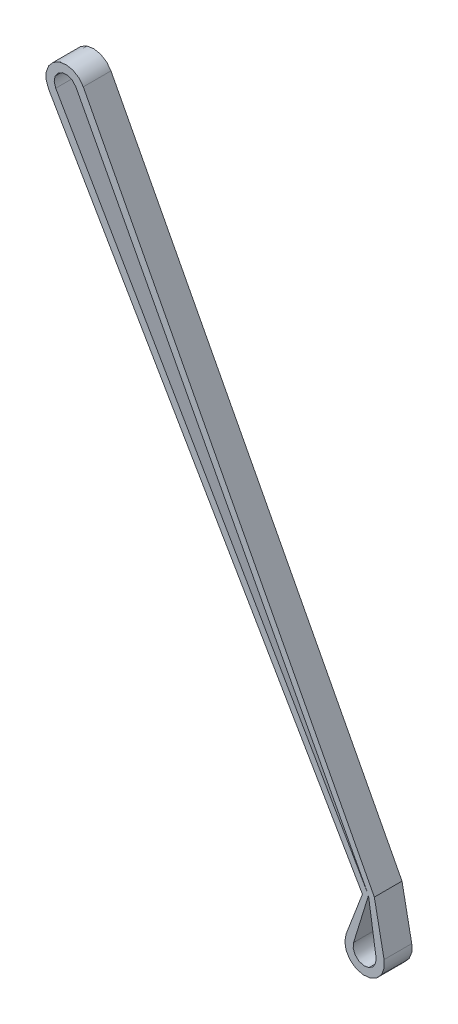
# Autodesk Inventor part: Angle Changer left band
Saved by Autodesk Inventor 2023.2 (Build 272271030, 271C)
## iProperties
Created: 2023-04-07
Part Number: Angle Changer left band
Material: Generic
Document SubType Name: Modeling
Designer: Main Account
Density: 1 g/cm^3
Appearance: Default
Author: Main Account
Autodesk Inventor part; units mm, degrees
ref_plane "YZ Plane" through (0, 0, 0) normal (1, 0, 0) x (0, 1, 0)
ref_plane "XZ Plane" through (0, 0, 0) normal (0, 1, 0) x (-1, 0, 0)
ref_plane "XY Plane" through (0, 0, 0) normal (0, 0, 1) x (1, 0, 0)
sketch "Sketch2" plane through (0, 0, 0) normal (0, 0, 1) x (1, 0, 0)
  circle A0 centre (4.0931, -20.1479) radius 2.1844 construction
  line L0 (57.7016, -119.5892) -> (56.531, -118.5169) construction
  circle A1 centre (58.0948, -128.5608) radius 2.1844 construction
  arc A2 (56.1046, -127.9465) -> (60.1543, -128.2505) centre (58.0948, -128.5608) ccw
  arc A3 (5.9348, -19.175) -> (2.2886, -21.1879) centre (4.0931, -20.1479) ccw
  arc A4 (54.75, -127.2766) -> (61.6095, -127.8658) centre (58.0948, -128.5608) ccw
  arc A5 (7.2676, -18.4867) -> (0.9949, -21.9473) centre (4.0931, -20.1479) ccw
  line L1 (54.75, -127.2766) -> (57.7016, -119.5892)
  line L2 (57.7016, -119.5892) -> (0.9949, -21.9473)
  line L3 (2.2886, -21.1879) -> (58.7941, -119.2338)
  line L4 (58.7941, -119.2338) -> (56.1046, -127.9465)
  line L5 (60.1543, -128.2505) -> (58.7957, -119.2343)
  line L6 (58.7957, -119.2343) -> (5.9348, -19.175)
  line L7 (7.2676, -18.4867) -> (59.8498, -118.9661)
  line L8 (59.8498, -118.9661) -> (61.6095, -127.8658)
  point P0 (0, 0)
  dimension "d17" = 4.1656
  dimension "d18" = 4.1656
  dimension "d19" = 1.5
  dimension "d20" = 1.5
  dimension "d21" = 1
  constraints: 16 end point, 10 point on circle, 8 tangent, 4 centre point, 2 coincident, 2 point on line
  measures "d17" diameter of A2
  measures "d18" diameter of A3
  measures "d19" radial gap between concentric circles of A2 A4
  measures "d20" radial gap between concentric circles of A3 A5
  measures "d21" distance from line of L0 L3.end
extrude "Extrusion2" add sketch "Sketch2" along normal blind 5
body "Solid2"
